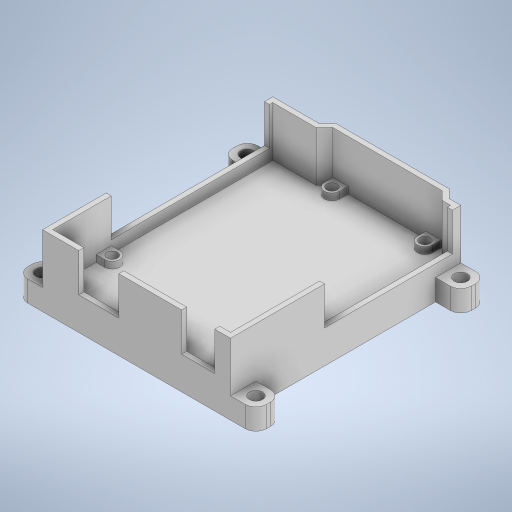
# Autodesk Inventor part: ArduinoCaseBottom
Saved by Autodesk Inventor 2024 (Build 280153000, 153)
## iProperties
Created: 2023-09-08
Part Number: ArduinoCaseBottom
Material: Generic
Document SubType Name: Modeling
Designer: 18179
Density: 1 g/cm^3
Appearance: Default
Autodesk Inventor part; units mm, degrees
(part 1 of 2)
ref_plane "YZ Plane" through (0, 0, 0) normal (1, 0, 0) x (0, 1, 0)
ref_plane "XZ Plane" through (0, 0, 0) normal (0, 1, 0) x (-1, 0, 0)
ref_plane "XY Plane" through (0, 0, 0) normal (0, 0, 1) x (1, 0, 0)
sketch "0" plane through (0, 0, 0) normal (0, 0, 1) x (1, 0, 0)
  line L0 (50.34, 19.545) -> (50.34, 17.135)
  line L1 (50.34, 17.135) -> (70.66, 17.135)
  line L2 (70.66, 17.135) -> (70.66, 19.545)
  line L3 (70.66, 19.545) -> (50.34, 19.545)
  line L4 (52.61, 19.34) -> (52.61, 17.34)
  line L5 (52.61, 17.34) -> (50.61, 17.34)
  line L6 (50.61, 17.34) -> (50.61, 19.34)
  line L7 (50.61, 19.34) -> (52.61, 19.34)
  line L8 (55.15, 17.34) -> (53.15, 17.34)
  line L9 (53.15, 17.34) -> (53.15, 19.34)
  line L10 (53.15, 19.34) -> (55.15, 19.34)
  line L11 (55.15, 19.34) -> (55.15, 17.34)
  line L12 (55.69, 17.34) -> (55.69, 19.34)
  line L13 (55.69, 19.34) -> (57.69, 19.34)
  line L14 (57.69, 19.34) -> (57.69, 17.34)
  line L15 (57.69, 17.34) -> (55.69, 17.34)
  line L16 (58.23, 17.34) -> (58.23, 19.34)
  line L17 (58.23, 19.34) -> (60.23, 19.34)
  line L18 (60.23, 19.34) -> (60.23, 17.34)
  line L19 (60.23, 17.34) -> (58.23, 17.34)
  line L20 (60.77, 17.34) -> (60.77, 19.34)
  line L21 (60.77, 19.34) -> (62.77, 19.34)
  line L22 (62.77, 19.34) -> (62.77, 17.34)
  line L23 (62.77, 17.34) -> (60.77, 17.34)
  line L24 (63.31, 17.34) -> (63.31, 19.34)
  line L25 (63.31, 19.34) -> (65.31, 19.34)
  line L26 (65.31, 19.34) -> (65.31, 17.34)
  line L27 (65.31, 17.34) -> (63.31, 17.34)
  line L28 (65.85, 17.34) -> (65.85, 19.34)
  line L29 (65.85, 19.34) -> (67.85, 19.34)
  line L30 (67.85, 19.34) -> (67.85, 17.34)
  line L31 (67.85, 17.34) -> (65.85, 17.34)
  line L32 (68.39, 17.34) -> (68.39, 19.34)
  line L33 (68.39, 19.34) -> (70.39, 19.34)
  line L34 (70.39, 19.34) -> (70.39, 17.34)
  line L35 (70.39, 17.34) -> (68.39, 17.34)
  line L36 (23.416, 19.545) -> (23.416, 17.135)
  line L37 (23.416, 17.135) -> (48.816, 17.135)
  line L38 (48.816, 17.135) -> (48.816, 19.545)
  line L39 (48.816, 19.545) -> (23.416, 19.545)
  line L40 (25.686, 19.34) -> (25.686, 17.34)
  line L41 (25.686, 17.34) -> (23.686, 17.34)
  line L42 (23.686, 17.34) -> (23.686, 19.34)
  line L43 (23.686, 19.34) -> (25.686, 19.34)
  line L44 (28.226, 17.34) -> (26.226, 17.34)
  line L45 (26.226, 17.34) -> (26.226, 19.34)
  line L46 (26.226, 19.34) -> (28.226, 19.34)
  line L47 (28.226, 19.34) -> (28.226, 17.34)
  line L48 (28.766, 17.34) -> (28.766, 19.34)
  line L49 (28.766, 19.34) -> (30.766, 19.34)
  line L50 (30.766, 19.34) -> (30.766, 17.34)
  line L51 (30.766, 17.34) -> (28.766, 17.34)
  line L52 (31.306, 17.34) -> (31.306, 19.34)
  line L53 (31.306, 19.34) -> (33.306, 19.34)
  line L54 (33.306, 19.34) -> (33.306, 17.34)
  line L55 (33.306, 17.34) -> (31.306, 17.34)
  line L56 (33.846, 17.34) -> (33.846, 19.34)
  line L57 (33.846, 19.34) -> (35.846, 19.34)
  line L58 (35.846, 19.34) -> (35.846, 17.34)
  line L59 (35.846, 17.34) -> (33.846, 17.34)
  line L60 (36.386, 17.34) -> (36.386, 19.34)
  line L61 (36.386, 19.34) -> (38.386, 19.34)
  line L62 (38.386, 19.34) -> (38.386, 17.34)
  line L63 (38.386, 17.34) -> (36.386, 17.34)
  line L64 (38.926, 17.34) -> (38.926, 19.34)
  line L65 (38.926, 19.34) -> (40.926, 19.34)
  line L66 (40.926, 19.34) -> (40.926, 17.34)
  line L67 (40.926, 17.34) -> (38.926, 17.34)
  line L68 (41.466, 17.34) -> (41.466, 19.34)
  line L69 (41.466, 19.34) -> (43.466, 19.34)
  line L70 (43.466, 19.34) -> (43.466, 17.34)
  line L71 (43.466, 17.34) -> (41.466, 17.34)
  line L72 (44.006, 17.34) -> (44.006, 19.34)
  line L73 (44.006, 19.34) -> (46.006, 19.34)
  line L74 (46.006, 19.34) -> (46.006, 17.34)
  line L75 (46.006, 17.34) -> (44.006, 17.34)
  line L76 (46.546, 17.34) -> (46.546, 19.34)
  line L77 (46.546, 19.34) -> (48.546, 19.34)
  line L78 (48.546, 19.34) -> (48.546, 17.34)
  line L79 (48.546, 17.34) -> (46.546, 17.34)
  line L80 (0, 0) -> (15.58, 0)
  line L81 (15.58, 0) -> (15.58, 11.12)
  line L82 (15.58, 11.12) -> (0, 11.12)
  line L83 (0, 11.12) -> (0, 0)
  line L84 (32.56, -28.715) -> (32.56, -31.125)
  line L85 (32.56, -31.125) -> (52.88, -31.125)
  line L86 (52.88, -31.125) -> (52.88, -28.715)
  line L87 (52.88, -28.715) -> (32.56, -28.715)
  line L88 (34.83, -28.92) -> (34.83, -30.92)
  line L89 (34.83, -30.92) -> (32.83, -30.92)
  line L90 (32.83, -30.92) -> (32.83, -28.92)
  line L91 (32.83, -28.92) -> (34.83, -28.92)
  line L92 (37.37, -30.92) -> (35.37, -30.92)
  line L93 (35.37, -30.92) -> (35.37, -28.92)
  line L94 (35.37, -28.92) -> (37.37, -28.92)
  line L95 (37.37, -28.92) -> (37.37, -30.92)
  line L96 (37.91, -30.92) -> (37.91, -28.92)
  line L97 (37.91, -28.92) -> (39.91, -28.92)
  line L98 (39.91, -28.92) -> (39.91, -30.92)
  line L99 (39.91, -30.92) -> (37.91, -30.92)
  line L100 (40.45, -30.92) -> (40.45, -28.92)
  line L101 (40.45, -28.92) -> (42.45, -28.92)
  line L102 (42.45, -28.92) -> (42.45, -30.92)
  line L103 (42.45, -30.92) -> (40.45, -30.92)
  line L104 (42.99, -30.92) -> (42.99, -28.92)
  line L105 (42.99, -28.92) -> (44.99, -28.92)
  line L106 (44.99, -28.92) -> (44.99, -30.92)
  line L107 (44.99, -30.92) -> (42.99, -30.92)
  line L108 (45.53, -30.92) -> (45.53, -28.92)
  line L109 (45.53, -28.92) -> (47.53, -28.92)
  line L110 (47.53, -28.92) -> (47.53, -30.92)
  line L111 (47.53, -30.92) -> (45.53, -30.92)
  line L112 (48.07, -30.92) -> (48.07, -28.92)
  line L113 (48.07, -28.92) -> (50.07, -28.92)
  line L114 (50.07, -28.92) -> (50.07, -30.92)
  line L115 (50.07, -30.92) -> (48.07, -30.92)
  line L116 (50.61, -30.92) -> (50.61, -28.92)
  line L117 (50.61, -28.92) -> (52.61, -28.92)
  line L118 (52.61, -28.92) -> (52.61, -30.92)
  line L119 (52.61, -30.92) -> (50.61, -30.92)
  line L120 (55.42, -28.715) -> (55.42, -31.125)
  line L121 (55.42, -31.125) -> (70.66, -31.125)
  line L122 (70.66, -31.125) -> (70.66, -28.715)
  line L123 (70.66, -28.715) -> (55.42, -28.715)
  line L124 (57.69, -28.92) -> (57.69, -30.92)
  line L125 (57.69, -30.92) -> (55.69, -30.92)
  line L126 (55.69, -30.92) -> (55.69, -28.92)
  line L127 (55.69, -28.92) -> (57.69, -28.92)
  line L128 (60.23, -30.92) -> (58.23, -30.92)
  line L129 (58.23, -30.92) -> (58.23, -28.92)
  line L130 (58.23, -28.92) -> (60.23, -28.92)
  line L131 (60.23, -28.92) -> (60.23, -30.92)
  line L132 (60.77, -30.92) -> (60.77, -28.92)
  line L133 (60.77, -28.92) -> (62.77, -28.92)
  line L134 (62.77, -28.92) -> (62.77, -30.92)
  line L135 (62.77, -30.92) -> (60.77, -30.92)
  line L136 (63.31, -30.92) -> (63.31, -28.92)
  line L137 (63.31, -28.92) -> (65.31, -28.92)
  line L138 (65.31, -28.92) -> (65.31, -30.92)
  line L139 (65.31, -30.92) -> (63.31, -30.92)
  line L140 (65.85, -30.92) -> (65.85, -28.92)
  line L141 (65.85, -28.92) -> (67.85, -28.92)
  line L142 (67.85, -28.92) -> (67.85, -30.92)
  line L143 (67.85, -30.92) -> (65.85, -30.92)
  line L144 (68.39, -30.92) -> (68.39, -28.92)
  line L145 (68.39, -28.92) -> (70.39, -28.92)
  line L146 (70.39, -28.92) -> (70.39, -30.92)
  line L147 (70.39, -30.92) -> (68.39, -30.92)
  arc A0 (68.8, -0.76) -> (68.3, -1.26) centre (68.8, -1.26) ccw
  line L148 (68.3, -1.26) -> (68.3, -2.8)
  arc A1 (68.3, -2.8) -> (68.8, -3.3) centre (68.8, -2.8) ccw
  line L149 (68.8, -3.3) -> (72.8, -3.3)
  arc A2 (72.8, -3.3) -> (73.3, -2.8) centre (72.8, -2.8) ccw
  line L150 (73.3, -2.8) -> (73.3, -1.26)
  arc A3 (73.3, -1.26) -> (72.8, -0.76) centre (72.8, -1.26) ccw
  line L151 (72.8, -0.76) -> (68.8, -0.76)
  line L152 (69.905, -2.405) -> (69.155, -2.405)
  line L153 (69.155, -2.405) -> (69.155, -1.655)
  line L154 (69.155, -1.655) -> (69.905, -1.655)
  line L155 (69.905, -1.655) -> (69.905, -2.405)
  line L156 (72.445, -2.405) -> (71.695, -2.405)
  line L157 (71.695, -2.405) -> (71.695, -1.655)
  line L158 (71.695, -1.655) -> (72.445, -1.655)
  line L159 (72.445, -1.655) -> (72.445, -2.405)
  arc A4 (68.8, -3.3) -> (68.3, -3.8) centre (68.8, -3.8) ccw
  line L160 (68.3, -3.8) -> (68.3, -5.34)
  arc A5 (68.3, -5.34) -> (68.8, -5.84) centre (68.8, -5.34) ccw
  line L161 (68.8, -5.84) -> (72.8, -5.84)
  arc A6 (72.8, -5.84) -> (73.3, -5.34) centre (72.8, -5.34) ccw
  line L162 (73.3, -5.34) -> (73.3, -3.8)
  arc A7 (73.3, -3.8) -> (72.8, -3.3) centre (72.8, -3.8) ccw
  line L163 (72.8, -3.3) -> (68.8, -3.3)
  line L164 (69.905, -4.945) -> (69.155, -4.945)
  line L165 (69.155, -4.945) -> (69.155, -4.195)
  line L166 (69.155, -4.195) -> (69.905, -4.195)
  line L167 (69.905, -4.195) -> (69.905, -4.945)
  line L168 (72.445, -4.945) -> (71.695, -4.945)
  line L169 (71.695, -4.945) -> (71.695, -4.195)
  line L170 (71.695, -4.195) -> (72.445, -4.195)
  line L171 (72.445, -4.195) -> (72.445, -4.945)
  arc A8 (68.8, -5.84) -> (68.3, -6.34) centre (68.8, -6.34) ccw
  line L172 (68.3, -6.34) -> (68.3, -7.88)
  arc A9 (68.3, -7.88) -> (68.8, -8.38) centre (68.8, -7.88) ccw
  line L173 (68.8, -8.38) -> (72.8, -8.38)
  arc A10 (72.8, -8.38) -> (73.3, -7.88) centre (72.8, -7.88) ccw
  line L174 (73.3, -7.88) -> (73.3, -6.34)
  arc A11 (73.3, -6.34) -> (72.8, -5.84) centre (72.8, -6.34) ccw
  line L175 (72.8, -5.84) -> (68.8, -5.84)
  line L176 (69.905, -7.485) -> (69.155, -7.485)
  line L177 (69.155, -7.485) -> (69.155, -6.735)
  line L178 (69.155, -6.735) -> (69.905, -6.735)
  line L179 (69.905, -6.735) -> (69.905, -7.485)
  line L180 (72.445, -7.485) -> (71.695, -7.485)
  line L181 (71.695, -7.485) -> (71.695, -6.735)
  line L182 (71.695, -6.735) -> (72.445, -6.735)
  line L183 (72.445, -6.735) -> (72.445, -7.485)
  arc A12 (20.37, 11.77) -> (20.87, 11.27) centre (20.87, 11.77) ccw
  line L184 (20.87, 11.27) -> (22.41, 11.27)
  arc A13 (22.41, 11.27) -> (22.91, 11.77) centre (22.41, 11.77) ccw
  line L185 (22.91, 11.77) -> (22.91, 15.77)
  arc A14 (22.91, 15.77) -> (22.41, 16.27) centre (22.41, 15.77) ccw
  line L186 (22.41, 16.27) -> (20.87, 16.27)
  arc A15 (20.87, 16.27) -> (20.37, 15.77) centre (20.87, 15.77) ccw
  line L187 (20.37, 15.77) -> (20.37, 11.77)
  line L188 (22.015, 12.875) -> (22.015, 12.125)
  line L189 (22.015, 12.125) -> (21.265, 12.125)
  line L190 (21.265, 12.125) -> (21.265, 12.875)
  line L191 (21.265, 12.875) -> (22.015, 12.875)
  line L192 (22.015, 15.415) -> (22.015, 14.665)
  line L193 (22.015, 14.665) -> (21.265, 14.665)
  line L194 (21.265, 14.665) -> (21.265, 15.415)
  line L195 (21.265, 15.415) -> (22.015, 15.415)
  arc A16 (25.45, 11.77) -> (25.95, 11.27) centre (25.95, 11.77) ccw
  line L196 (25.95, 11.27) -> (27.49, 11.27)
  arc A17 (27.49, 11.27) -> (27.99, 11.77) centre (27.49, 11.77) ccw
  line L197 (27.99, 11.77) -> (27.99, 15.77)
  arc A18 (27.99, 15.77) -> (27.49, 16.27) centre (27.49, 15.77) ccw
  line L198 (27.49, 16.27) -> (25.95, 16.27)
  arc A19 (25.95, 16.27) -> (25.45, 15.77) centre (25.95, 15.77) ccw
  line L199 (25.45, 15.77) -> (25.45, 11.77)
  line L200 (27.095, 12.875) -> (27.095, 12.125)
  line L201 (27.095, 12.125) -> (26.345, 12.125)
  line L202 (26.345, 12.125) -> (26.345, 12.875)
  line L203 (26.345, 12.875) -> (27.095, 12.875)
  line L204 (27.095, 15.415) -> (27.095, 14.665)
  line L205 (27.095, 14.665) -> (26.345, 14.665)
  line L206 (26.345, 14.665) -> (26.345, 15.415)
  line L207 (26.345, 15.415) -> (27.095, 15.415)
  arc A20 (22.91, 11.77) -> (23.41, 11.27) centre (23.41, 11.77) ccw
  line L208 (23.41, 11.27) -> (24.95, 11.27)
  arc A21 (24.95, 11.27) -> (25.45, 11.77) centre (24.95, 11.77) ccw
  line L209 (25.45, 11.77) -> (25.45, 15.77)
  arc A22 (25.45, 15.77) -> (24.95, 16.27) centre (24.95, 15.77) ccw
  line L210 (24.95, 16.27) -> (23.41, 16.27)
  arc A23 (23.41, 16.27) -> (22.91, 15.77) centre (23.41, 15.77) ccw
  line L211 (22.91, 15.77) -> (22.91, 11.77)
  line L212 (24.555, 12.875) -> (24.555, 12.125)
  line L213 (24.555, 12.125) -> (23.805, 12.125)
  line L214 (23.805, 12.125) -> (23.805, 12.875)
  line L215 (23.805, 12.875) -> (24.555, 12.875)
  line L216 (24.555, 15.415) -> (24.555, 14.665)
  line L217 (24.555, 14.665) -> (23.805, 14.665)
  line L218 (23.805, 14.665) -> (23.805, 15.415)
  line L219 (23.805, 15.415) -> (24.555, 15.415)
  line L220 (64.91, 3.516) -> (64.91, 4.716)
  line L221 (64.91, 4.716) -> (63.71, 4.716)
  line L222 (63.71, 4.716) -> (63.71, 3.516)
  line L223 (63.71, 3.516) -> (64.91, 3.516)
  line L224 (34.43, 8.977) -> (34.43, 10.177)
  line L225 (34.43, 10.177) -> (33.23, 10.177)
  line L226 (33.23, 10.177) -> (33.23, 8.977)
  line L227 (33.23, 8.977) -> (34.43, 8.977)
  line L228 (34.43, 3.77) -> (34.43, 4.97)
  line L229 (34.43, 4.97) -> (33.23, 4.97)
  line L230 (33.23, 4.97) -> (33.23, 3.77)
  line L231 (33.23, 3.77) -> (34.43, 3.77)
  line L232 (34.43, 1.23) -> (34.43, 2.43)
  line L233 (34.43, 2.43) -> (33.23, 2.43)
  line L234 (33.23, 2.43) -> (33.23, 1.23)
  line L235 (33.23, 1.23) -> (34.43, 1.23)
  line L236 (5.89, -32.46) -> (71.93, -32.46)
  line L237 (71.93, -32.46) -> (71.93, -29.92)
  line L238 (71.93, -29.92) -> (74.47, -27.38)
  line L239 (74.47, -27.38) -> (74.47, 5.386)
  line L240 (74.47, 5.386) -> (71.93, 7.926)
  line L241 (71.93, 7.926) -> (71.93, 20.88)
  line L242 (71.93, 20.88) -> (5.89, 20.88)
  line L243 (5.89, 20.88) -> (5.89, -32.46)
  line L244 (15.985, -20.785) -> (7.485, -20.785)
  line L245 (7.485, -20.785) -> (7.485, -20.285)
  line L246 (7.485, -20.285) -> (3.985, -20.285)
  line L247 (3.985, -29.285) -> (7.485, -29.285)
  line L248 (7.485, -29.285) -> (7.485, -28.785)
  line L249 (7.485, -28.785) -> (15.985, -28.785)
  line L250 (15.48, 11.58) -> (0.1, 11.58)
  line L251 (16.04, 0) -> (16.04, 11.12)
  line L252 (0.1, -0.46) -> (15.48, -0.46)
  line L253 (-0.46, 0) -> (-0.46, 11.12)
  circle A24 centre (12.24, 16.943) radius 1.5
  line L254 (17.685, -20.785) -> (17.685, -28.785)
  line L255 (3.985, -20.785) -> (3.985, -28.785)
  circle A25 centre (21.13, 18.34) radius 1.5875
  circle A26 centre (19.86, -29.92) radius 1.5875
  circle A27 centre (71.93, 3.1) radius 1.5875
  circle A28 centre (71.93, -24.84) radius 1.5875
  circle A29 centre (68.755, -19.887) radius 0.4
  circle A30 centre (68.755, -12.267) radius 0.4
  circle A31 centre (66.215, -19.887) radius 0.4
  circle A32 centre (66.215, -12.267) radius 0.4
  circle A33 centre (63.675, -19.887) radius 0.4
  circle A34 centre (63.675, -12.267) radius 0.4
  circle A35 centre (61.135, -19.887) radius 0.4
  circle A36 centre (61.135, -12.267) radius 0.4
  circle A37 centre (58.595, -19.887) radius 0.4
  circle A38 centre (58.595, -12.267) radius 0.4
  circle A39 centre (56.055, -19.887) radius 0.4
  circle A40 centre (56.055, -12.267) radius 0.4
  circle A41 centre (53.515, -19.887) radius 0.4
  circle A42 centre (53.515, -12.267) radius 0.4
  circle A43 centre (50.975, -19.887) radius 0.4
  circle A44 centre (50.975, -12.267) radius 0.4
  circle A45 centre (48.435, -19.887) radius 0.4
  circle A46 centre (48.435, -12.267) radius 0.4
  circle A47 centre (45.895, -19.887) radius 0.4
  circle A48 centre (45.895, -12.267) radius 0.4
  circle A49 centre (43.355, -19.887) radius 0.4
  circle A50 centre (43.355, -12.267) radius 0.4
  circle A51 centre (40.815, -19.887) radius 0.4
  circle A52 centre (40.815, -12.267) radius 0.4
  circle A53 centre (38.275, -19.887) radius 0.4
  circle A54 centre (38.275, -12.267) radius 0.4
  circle A55 centre (35.735, -19.887) radius 0.4
  circle A56 centre (35.735, -12.267) radius 0.4
  circle A57 centre (22.273, -6.298) radius 0.5
  circle A58 centre (27.353, -6.298) radius 0.5
  circle A59 centre (24.178, 7.418) radius 0.4
  circle A60 centre (26.718, 7.418) radius 0.4
  circle A61 centre (26.718, 9.958) radius 0.4
  circle A62 centre (24.178, 9.958) radius 0.4
  circle A63 centre (21.638, 12.498) radius 0.4
  circle A64 centre (24.178, 12.498) radius 0.4
  circle A65 centre (26.718, 12.498) radius 0.4
  circle A66 centre (26.718, 15.038) radius 0.4
  circle A67 centre (24.178, 15.038) radius 0.4
  circle A68 centre (21.638, 15.038) radius 0.4
  circle A69 centre (69.53, -2.03) radius 0.4
  circle A70 centre (69.53, -4.57) radius 0.4
  circle A71 centre (69.53, -7.11) radius 0.4
  circle A72 centre (72.07, -7.11) radius 0.4
  circle A73 centre (72.07, -4.57) radius 0.4
  circle A74 centre (72.07, -2.03) radius 0.4
  circle A75 centre (54.15, 18.34) radius 0.4
  circle A76 centre (27.226, 18.34) radius 0.4
  circle A77 centre (51.61, 18.34) radius 0.4
  circle A78 centre (36.37, -29.92) radius 0.4
  circle A79 centre (24.686, 18.34) radius 0.4
  circle A80 centre (33.83, -29.92) radius 0.4
  circle A81 centre (21.13, 18.34) radius 1.5875
  circle A82 centre (19.86, -29.92) radius 1.5875
  circle A83 centre (71.93, 3.1) radius 1.5875
  circle A84 centre (71.93, -24.84) radius 1.5875
  circle A85 centre (38.91, -29.92) radius 0.4
  circle A86 centre (41.45, -29.92) radius 0.4
  circle A87 centre (43.99, -29.92) radius 0.4
  circle A88 centre (46.53, -29.92) radius 0.4
  circle A89 centre (49.07, -29.92) radius 0.4
  circle A90 centre (51.61, -29.92) radius 0.4
  circle A91 centre (56.69, -29.92) radius 0.4
  circle A92 centre (59.23, -29.92) radius 0.4
  circle A93 centre (61.77, -29.92) radius 0.4
  circle A94 centre (64.31, -29.92) radius 0.4
  circle A95 centre (66.85, -29.92) radius 0.4
  circle A96 centre (69.39, -29.92) radius 0.4
  circle A97 centre (29.766, 18.34) radius 0.4
  circle A98 centre (32.306, 18.34) radius 0.4
  circle A99 centre (34.846, 18.34) radius 0.4
  circle A100 centre (37.386, 18.34) radius 0.4
  circle A101 centre (39.926, 18.34) radius 0.4
  circle A102 centre (42.466, 18.34) radius 0.4
  circle A103 centre (45.006, 18.34) radius 0.4
  circle A104 centre (47.546, 18.34) radius 0.4
  circle A105 centre (56.69, 18.34) radius 0.4
  circle A106 centre (59.23, 18.34) radius 0.4
  circle A107 centre (61.77, 18.34) radius 0.4
  circle A108 centre (64.31, 18.34) radius 0.4
  circle A109 centre (66.85, 18.34) radius 0.4
  circle A110 centre (69.39, 18.34) radius 0.4
  line L256 (4.3025, 20.88) -> (4.3025, -32.46)
  line L257 (71.93, 22.4675) -> (5.89, 22.4675)
  line L258 (73.5175, 7.926) -> (73.5175, 20.88)
  line L259 (75.5925, 6.5085) -> (73.0525, 9.0485)
  line L260 (76.0575, -27.38) -> (76.0575, 5.386)
  line L261 (73.0525, -31.0425) -> (75.5925, -28.5025)
  line L262 (73.5175, -32.46) -> (73.5175, -29.92)
  line L263 (5.89, -34.0475) -> (71.93, -34.0475)
  line L264 (4.3025, 20.88) -> (4.3025, 22.4675)
  line L265 (4.3025, 22.4675) -> (5.89, 22.4675)
  line L266 (71.93, 22.4675) -> (73.5175, 22.4675)
  line L267 (73.5175, 22.4675) -> (73.5175, 20.88)
  line L268 (76.0575, 5.386) -> (76.0575, 7.7785)
  line L269 (75.5925, 6.5085) -> (76.0575, 6.0436)
  line L270 (71.93, -34.0475) -> (73.5175, -34.0475)
  line L271 (73.5175, -34.0475) -> (73.5175, -32.46)
  line L272 (75.5925, -28.5025) -> (76.6188, -27.4763)
  line L273 (76.0575, -27.38) -> (76.1056, -27.9894)
  line L274 (4.3025, -32.46) -> (4.3025, -34.0475)
  line L275 (4.3025, -34.0475) -> (5.89, -34.0475)
  line L276 (4.3025, 22.4675) -> (11.9225, 22.4675)
  line L277 (11.9225, 22.4675) -> (11.9225, 26.9125)
  line L278 (8.7475, 30.0875) -> (7.4775, 30.0875)
  line L279 (4.3025, 26.9125) -> (4.3025, 22.4675)
  circle A111 centre (8.1125, 26.2775) radius 2
  line L280 (73.5175, 22.4675) -> (65.8975, 22.4675)
  line L281 (65.8975, 22.4675) -> (65.8975, 26.9125)
  line L282 (69.0725, 30.0875) -> (70.3425, 30.0875)
  line L283 (73.5175, 26.9125) -> (73.5175, 22.4675)
  line L284 (4.3025, -34.0475) -> (11.9225, -34.0475)
  line L285 (11.9225, -34.0475) -> (11.9225, -38.4925)
  line L286 (8.7475, -41.6675) -> (7.4775, -41.6675)
  line L287 (4.3025, -38.4925) -> (4.3025, -34.0475)
  line L288 (73.5175, -34.0475) -> (65.8975, -34.0475)
  line L289 (65.8975, -34.0475) -> (65.8975, -38.4925)
  line L290 (69.0725, -41.6675) -> (70.3425, -41.6675)
  line L291 (73.5175, -38.4925) -> (73.5175, -34.0475)
  circle A112 centre (8.1125, -37.8575) radius 2
  circle A113 centre (69.7075, -37.8575) radius 2
  circle A114 centre (69.7075, 26.2775) radius 2
  arc A115 (7.4775, 30.0875) -> (4.3025, 26.9125) centre (7.4775, 26.9125) ccw
  arc A116 (11.9225, 26.9125) -> (8.7475, 30.0875) centre (8.7475, 26.9125) ccw
  arc A117 (69.0725, 30.0875) -> (65.8975, 26.9125) centre (69.0725, 26.9125) ccw
  arc A118 (73.5175, 26.9125) -> (70.3425, 30.0875) centre (70.3425, 26.9125) ccw
  arc A119 (70.3425, -41.6675) -> (73.5175, -38.4925) centre (70.3425, -38.4925) ccw
  arc A120 (65.8975, -38.4925) -> (69.0725, -41.6675) centre (69.0725, -38.4925) ccw
  arc A121 (8.7475, -41.6675) -> (11.9225, -38.4925) centre (8.7475, -38.4925) ccw
  arc A122 (4.3025, -38.4925) -> (7.4775, -41.6675) centre (7.4775, -38.4925) ccw
  point P0 (11.9225, 30.0875)
  point P1 (4.3025, 30.0875)
  point P2 (65.8975, 30.0875)
  point P3 (73.5175, 30.0875)
  point P4 (11.9225, -41.6675)
  point P5 (4.3025, -41.6675)
  point P6 (65.8975, -41.6675)
  point P7 (73.5175, -41.6675)
  point P8 (4.3025, 11.12)
  point P9 (4.3025, 0)
  point P10 (5.89, 0)
  point P11 (5.89, 11.12)
  point P12 (4.3025, 11.58)
  point P13 (5.89, 11.58)
  point P14 (74.47, 5.386)
  point P15 (5.89, -32.46)
  point P16 (5.89, -0.46)
  point P17 (4.3025, -0.46)
  point P18 (73.5175, -30.5776)
  point P19 (73.5175, 8.5836)
  point P20 (4.3025, -20.285)
  point P21 (4.3025, -29.285)
  point P22 (5.89, -29.285)
  point P23 (5.89, -20.285)
  point P24 (69.905, -4.7092)
  point P25 (69.6692, -4.945)
  point P26 (69.3908, -4.945)
  point P27 (69.155, -4.7092)
  point P28 (69.155, -4.4308)
  point P29 (69.3908, -4.195)
  point P30 (69.6692, -4.195)
  point P31 (69.905, -4.4308)
  point P32 (72.445, -4.7092)
  point P33 (72.2092, -4.945)
  point P34 (71.9308, -4.945)
  point P35 (71.695, -4.7092)
  point P36 (71.695, -4.4308)
  point P37 (71.9308, -4.195)
  point P38 (72.2092, -4.195)
  point P39 (72.445, -4.4308)
  point P40 (69.905, -7.2492)
  point P41 (69.6692, -7.485)
  point P42 (69.3908, -7.485)
  point P43 (69.155, -7.2492)
  point P44 (69.155, -6.9708)
  point P45 (69.3908, -6.735)
  point P46 (69.6692, -6.735)
  point P47 (69.905, -6.9708)
  point P48 (68.8, -0.76)
  point P49 (68.3, -6.34)
  point P50 (68.8, -8.38)
  point P51 (69.905, -2.1692)
  point P52 (69.6692, -2.405)
  point P53 (69.3908, -2.405)
  point P54 (69.155, -2.1692)
  point P55 (69.155, -1.8908)
  point P56 (69.3908, -1.655)
  point P57 (69.6692, -1.655)
  point P58 (69.905, -1.8908)
  point P59 (72.445, -2.1692)
  point P60 (72.2092, -2.405)
  point P61 (71.9308, -2.405)
  point P62 (71.695, -2.1692)
  point P63 (71.695, -1.8908)
  point P64 (71.9308, -1.655)
  point P65 (72.2092, -1.655)
  point P66 (72.445, -1.8908)
  point P67 (24.555, 12.3643)
  point P68 (24.3225, 12.125)
  point P69 (24.0335, 12.125)
  point P70 (23.805, 12.3535)
  point P71 (23.805, 12.6425)
  point P72 (24.0443, 12.875)
  point P73 (24.3117, 12.875)
  point P74 (24.555, 12.6317)
  point P75 (24.555, 14.9043)
  point P76 (24.3225, 14.665)
  point P77 (24.0335, 14.665)
  point P78 (23.805, 14.8935)
  point P79 (23.805, 15.1825)
  point P80 (24.0443, 15.415)
  point P81 (24.3117, 15.415)
  point P82 (24.555, 15.1717)
  point P83 (27.095, 12.3643)
  point P84 (26.8625, 12.125)
  point P85 (26.5735, 12.125)
  point P86 (26.345, 12.3535)
  point P87 (26.345, 12.6425)
  point P88 (26.5843, 12.875)
  point P89 (26.8517, 12.875)
  point P90 (27.095, 12.6317)
  point P91 (27.095, 14.9043)
  point P92 (26.8625, 14.665)
  point P93 (26.5735, 14.665)
  point P94 (26.345, 14.8935)
  point P95 (26.345, 15.1825)
  point P96 (26.5843, 15.415)
  point P97 (26.8517, 15.415)
  point P98 (27.095, 15.1717)
  point P99 (22.41, 16.27)
  point P100 (20.37, 11.77)
  point P101 (23.41, 11.27)
  point P102 (27.49, 16.27)
  point P103 (24.95, 16.27)
  point P104 (22.015, 12.3643)
  point P105 (21.7825, 12.125)
  point P106 (21.4935, 12.125)
  point P107 (21.265, 12.3535)
  point P108 (21.265, 12.6425)
  point P109 (21.5043, 12.875)
  point P110 (21.7717, 12.875)
  point P111 (22.015, 12.6317)
  point P112 (22.015, 14.9043)
  point P113 (21.7825, 14.665)
  point P114 (21.4935, 14.665)
  point P115 (21.265, 14.8935)
  point P116 (21.265, 15.1825)
  point P117 (21.5043, 15.415)
  point P118 (21.7717, 15.415)
  point P119 (22.015, 15.1717)
  dimension "d0" = 1.5875
  dimension "d1" = 1.5875
  dimension "d2" = 1.5875
  dimension "d3" = 1.5875
  dimension "d4" = 1.5875
  dimension "d5" = 1.5875
  dimension "d6" = 1.5875
  dimension "d7" = 1.5875
  dimension "d8" = 7.62
  dimension "d9" = 7.62
  dimension "d10" = 4
  dimension "d11" = 7.62
  dimension "d12" = 7.62
  dimension "d13" = 7.62
  dimension "d14" = 7.62
  dimension "d15" = 7.62
  dimension "d16" = 7.62
  dimension "d17" = 4
  dimension "d18" = 4
  dimension "d19" = 4
  dimension "d20" = 3.175
  constraints: 584 end point, 131 horizontal, 131 vertical, 123 centre point, 64 point on circle, 18 point on line, 16 parallel, 16 tangent, 9 perpendicular, 7 equal radius, 1 midpoint, 784 other
  measures "d0" distance between parallel lines of L243 L256
  measures "d1" distance between parallel lines of L242 L257
  measures "d2" distance between parallel lines of L241 L258
  measures "d3" distance between parallel lines of L240 L259
  measures "d4" distance between parallel lines of L239 L260
  measures "d5" distance between parallel lines of L238 L261
  measures "d6" distance between parallel lines of L237 L262
  measures "d7" distance between parallel lines of L236 L263
  measures "d8" distance of point (4.302, 30.087) point (11.922, 30.087)
  measures "d9" distance of point (11.922, 30.087) L276.end
  measures "d10" diameter of A111
  measures "d11" distance of point (65.897, 30.087) point (73.517, 30.087)
  measures "d12" distance of L280.end point (65.897, 30.087)
  measures "d13" distance of point (11.922, -41.668) point (4.302, -41.668)
  measures "d14" distance of L284.end point (11.922, -41.668)
  measures "d15" distance of point (73.517, -41.668) point (65.897, -41.668)
  measures "d16" distance of point (65.897, -41.668) L288.end
  measures "d17" diameter of A112
  measures "d18" diameter of A113
  measures "d19" diameter of A114
  measures "d20" radius of A115
extrude "Extrusion1" add sketch "0" along normal blind 3.175 contours L256 L82 L243 L80 | L252 L243 L246 L256 | L256 L264 L265 L257 L266 L267 L258 L259 L269 L268 L260 L273 L272 L261 L262 L271 L270 L263 L275 L274 L247 L243 L236 L237 L238 L239 L240 L241 L242 L250 | L246 L243 L247 L256 | L279 A115 L278 A116 L277 L257 L265 | L275 L263 L285 A121 L286 A122 L287 | L281 A117 L282 A118 L283 L266 L257 | L263 L270 L291 A119 L290 A120 L289
extrude "Extrusion2" add sketch "0" along normal blind 3.175 contours L80 L243 L252 L256 | L256 L250 L243 L82
sketch "Sketch3" plane through (0, 0, 3.175) normal (0, 0, 1) x (1, 0, 0)
  line L0 (4.3025, 26.9125) -> (4.3025, -38.4925) projected
  arc A0 (4.3025, -38.4925) -> (7.4775, -41.6675) centre (7.4775, -38.4925) ccw projected
  line L1 (7.4775, -41.6675) -> (8.7475, -41.6675) projected
  arc A1 (8.7475, -41.6675) -> (11.9225, -38.4925) centre (8.7475, -38.4925) ccw projected
  line L2 (11.9225, -38.4925) -> (11.9225, -34.0475) projected
  line L3 (11.9225, -34.0475) -> (65.8975, -34.0475) projected
  line L4 (65.8975, -34.0475) -> (65.8975, -38.4925) projected
  arc A2 (65.8975, -38.4925) -> (69.0725, -41.6675) centre (69.0725, -38.4925) ccw projected
  line L5 (69.0725, -41.6675) -> (70.3425, -41.6675) projected
  arc A3 (70.3425, -41.6675) -> (73.5175, -38.4925) centre (70.3425, -38.4925) ccw projected
  line L6 (73.5175, -38.4925) -> (73.5175, -30.5776) projected
  line L7 (73.5175, -30.5776) -> (76.1056, -27.9894) projected
  line L8 (76.1056, -27.9894) -> (76.0575, -27.38) projected
  line L9 (76.0575, -27.38) -> (76.0575, 6.0436) projected
  line L10 (76.0575, 6.0436) -> (73.5175, 8.5836) projected
  line L11 (73.5175, 8.5836) -> (73.5175, 26.9125) projected
  arc A4 (73.5175, 26.9125) -> (70.3425, 30.0875) centre (70.3425, 26.9125) ccw projected
  line L12 (70.3425, 30.0875) -> (69.0725, 30.0875) projected
  arc A5 (69.0725, 30.0875) -> (65.8975, 26.9125) centre (69.0725, 26.9125) ccw projected
  line L13 (65.8975, 26.9125) -> (65.8975, 22.4675) projected
  line L14 (65.8975, 22.4675) -> (11.9225, 22.4675) projected
  line L15 (11.9225, 22.4675) -> (11.9225, 26.9125) projected
  arc A6 (11.9225, 26.9125) -> (8.7475, 30.0875) centre (8.7475, 26.9125) ccw projected
  line L16 (8.7475, 30.0875) -> (7.4775, 30.0875) projected
  arc A7 (7.4775, 30.0875) -> (4.3025, 26.9125) centre (7.4775, 26.9125) ccw projected
  circle A8 centre (8.1125, 26.2775) radius 2 projected
  circle A9 centre (69.7075, 26.2775) radius 2 projected
  circle A10 centre (69.7075, -37.8575) radius 2 projected
  circle A11 centre (8.1125, -37.8575) radius 2 projected
  line L17 (5.89, -32.46) -> (5.89, 20.88) projected
  line L18 (5.89, 20.88) -> (71.93, 20.88) projected
  line L19 (71.93, 20.88) -> (71.93, 7.926) projected
  line L20 (71.93, 7.926) -> (74.47, 5.386) projected
  line L21 (74.47, 5.386) -> (74.47, -27.38) projected
  line L22 (74.47, -27.38) -> (71.93, -29.92) projected
  line L23 (71.93, -29.92) -> (71.93, -32.46) projected
  line L24 (71.93, -32.46) -> (5.89, -32.46) projected
  point P0 (0, 0)
extrude "Extrusion3" add sketch "Sketch3" along normal blind 3.175 contours A7 L16 A6 L15 L14 L13 A5 L12 A4 L11 L10 L9 L8 L7 L6 A3 L5 A2 L4 L3 L2 A1 L1 A0 L0 | L17 L18 L19 L20 L21 L22 L23 L24
extrude "Extrusion4" cut sketch "0" along normal through all contours A25 | A26 | A27 | A28
sketch "Sketch4" plane through (0, 0, 6.35) normal (0, 0, 1) x (1, 0, 0)
  circle A0 centre (71.93, 3.1) radius 1.5875 projected
  circle A1 centre (21.13, 18.34) radius 1.5875 projected
  circle A2 centre (71.93, -24.84) radius 1.5875 projected
  circle A3 centre (19.86, -29.92) radius 1.5875 projected
  arc A4 (4.3025, -38.4925) -> (7.4775, -41.6675) centre (7.4775, -38.4925) ccw projected
  line L0 (7.4775, -41.6675) -> (8.7475, -41.6675) projected
  arc A5 (8.7475, -41.6675) -> (11.9225, -38.4925) centre (8.7475, -38.4925) ccw projected
  line L1 (11.9225, -38.4925) -> (11.9225, -34.0475) projected
  line L2 (11.9225, -34.0475) -> (65.8975, -34.0475) projected
  line L3 (65.8975, -34.0475) -> (65.8975, -38.4925) projected
  arc A6 (65.8975, -38.4925) -> (69.0725, -41.6675) centre (69.0725, -38.4925) ccw projected
  line L4 (69.0725, -41.6675) -> (70.3425, -41.6675) projected
  arc A7 (70.3425, -41.6675) -> (73.5175, -38.4925) centre (70.3425, -38.4925) ccw projected
  line L5 (73.5175, -38.4925) -> (73.5175, -30.5776) projected
  line L6 (73.5175, -30.5776) -> (76.1056, -27.9894) projected
  line L7 (76.1056, -27.9894) -> (76.0575, -27.38) projected
  line L8 (76.0575, -27.38) -> (76.0575, 6.0436) projected
  line L9 (76.0575, 6.0436) -> (73.5175, 8.5836) projected
  line L10 (73.5175, 8.5836) -> (73.5175, 26.9125) projected
  arc A8 (73.5175, 26.9125) -> (70.3425, 30.0875) centre (70.3425, 26.9125) ccw projected
  line L11 (70.3425, 30.0875) -> (69.0725, 30.0875) projected
  arc A9 (69.0725, 30.0875) -> (65.8975, 26.9125) centre (69.0725, 26.9125) ccw projected
  line L12 (65.8975, 26.9125) -> (65.8975, 22.4675) projected
  line L13 (65.8975, 22.4675) -> (11.9225, 22.4675) projected
  line L14 (11.9225, 22.4675) -> (11.9225, 26.9125) projected
  arc A10 (11.9225, 26.9125) -> (8.7475, 30.0875) centre (8.7475, 26.9125) ccw projected
  line L15 (8.7475, 30.0875) -> (7.4775, 30.0875) projected
  arc A11 (7.4775, 30.0875) -> (4.3025, 26.9125) centre (7.4775, 26.9125) ccw projected
  line L16 (4.3025, 26.9125) -> (4.3025, -38.4925) projected
  circle A12 centre (8.1125, -37.8575) radius 2 projected
  circle A13 centre (69.7075, -37.8575) radius 2 projected
  circle A14 centre (69.7075, 26.2775) radius 2 projected
  circle A15 centre (8.1125, 26.2775) radius 2 projected
  line L17 (10.3985, 20.9435) -> (67.4215, 20.9435)
  line L18 (67.4215, 20.9435) -> (67.4215, 26.9125)
  arc A16 (69.0725, 28.5635) -> (67.4215, 26.9125) centre (69.0725, 26.9125) ccw
  line L19 (69.0725, 28.5635) -> (70.3425, 28.5635)
  arc A17 (71.9935, 26.9125) -> (70.3425, 28.5635) centre (70.3425, 26.9125) ccw
  line L20 (71.9935, 26.9125) -> (71.9935, 7.9523)
  line L21 (71.9935, 7.9523) -> (74.5335, 5.4123)
  line L22 (74.5335, 5.4123) -> (74.5335, -27.4063)
  line L23 (74.5335, -27.4063) -> (71.9935, -29.9463)
  line L24 (71.9935, -29.9463) -> (71.9935, -38.4925)
  arc A18 (70.3425, -40.1435) -> (71.9935, -38.4925) centre (70.3425, -38.4925) ccw
  line L25 (70.3425, -40.1435) -> (69.0725, -40.1435)
  arc A19 (67.4215, -38.4925) -> (69.0725, -40.1435) centre (69.0725, -38.4925) ccw
  line L26 (67.4215, -38.4925) -> (67.4215, -32.5235)
  line L27 (67.4215, -32.5235) -> (10.3985, -32.5235)
  line L28 (10.3985, -32.5235) -> (10.3985, -38.4925)
  arc A20 (8.7475, -40.1435) -> (10.3985, -38.4925) centre (8.7475, -38.4925) ccw
  line L29 (8.7475, -40.1435) -> (7.4775, -40.1435)
  arc A21 (5.8265, -38.4925) -> (7.4775, -40.1435) centre (7.4775, -38.4925) ccw
  line L30 (5.8265, -38.4925) -> (5.8265, 26.9125)
  arc A22 (7.4775, 28.5635) -> (5.8265, 26.9125) centre (7.4775, 26.9125) ccw
  line L31 (7.4775, 28.5635) -> (8.7475, 28.5635)
  arc A23 (10.3985, 26.9125) -> (8.7475, 28.5635) centre (8.7475, 26.9125) ccw
  line L32 (10.3985, 26.9125) -> (10.3985, 20.9435)
  line L33 (10.3985, 20.9435) -> (5.8265, 20.9435)
  line L34 (67.4215, 20.9435) -> (71.9935, 20.9435)
  line L35 (67.4215, -32.5235) -> (71.9935, -32.5235)
  line L36 (10.3985, -32.5235) -> (5.8265, -32.5235)
  line L37 (65.8975, 22.4675) -> (73.5175, 22.4675)
  line L38 (11.9225, 22.4675) -> (4.3025, 22.4675)
  line L39 (11.9225, -34.0475) -> (4.3025, -34.0475)
  line L40 (65.8975, -34.0475) -> (73.5175, -34.0475)
  point P0 (0, 0)
  dimension "d29" = 1.524
  constraints: 48 end point, 16 point on circle, 12 point on line, 8 centre point, 4 perpendicular, 23 other
  measures "d29" distance between parallel lines of L13 L17
extrude "Extrusion5" add sketch "Sketch4" along normal blind 15 contours L16 L38 L30 L39 | L30 L36 L28 L39 | L38 L32 L33 L30 | L28 L27 L26 L40 L2 L39 | L38 L13 L37 L18 L17 L32 | L35 L24 L40 L26 | L18 L37 L20 L34 | L24 L23 L22 L21 L20 L37 L10 L9 L8 L7 L6 L5 L40
extrude "Extrusion6" cut sketch "0" along normal through all contours L256 L82 L243 L80 | L246 L243 L247 L256
sketch "Sketch5" plane through (0, 0, 6.35) normal (0, 0, 1) x (1, 0, 0)
  circle A0 centre (19.86, -29.92) radius 1.5875 projected
  circle A1 centre (71.93, -24.84) radius 1.5875 projected
  circle A2 centre (21.13, 18.34) radius 1.5875 projected
  circle A3 centre (71.93, 3.1) radius 1.5875 projected
  line L0 (5.8265, 11.12) -> (5.89, 11.12) projected
  line L1 (5.89, 11.12) -> (5.89, 0) projected
  line L2 (5.89, 0) -> (5.8265, 0) projected
  line L3 (5.8265, 20.9435) -> (5.8265, 11.12) projected
  line L4 (5.8265, -20.285) -> (5.89, -20.285) projected
  line L5 (5.89, -20.285) -> (5.89, -29.285) projected
  line L6 (5.89, -29.285) -> (5.8265, -29.285) projected
  line L7 (5.8265, -29.285) -> (5.8265, -32.5235) projected
  line L8 (5.8265, -32.5235) -> (71.9935, -32.5235) projected
  line L9 (71.9935, -32.5235) -> (71.9935, -29.9463) projected
  line L10 (71.9935, -29.9463) -> (74.5335, -27.4063) projected
  line L11 (74.5335, -27.4063) -> (74.5335, 5.4123) projected
  line L12 (74.5335, 5.4123) -> (71.9935, 7.9523) projected
  line L13 (71.9935, 7.9523) -> (71.9935, 20.9435) projected
  line L14 (71.9935, 20.9435) -> (5.8265, 20.9435) projected
  line L15 (5.8265, 0) -> (5.8265, -20.285) projected
  circle A4 centre (21.13, 18.34) radius 2.286
  circle A5 centre (71.93, 3.1) radius 2.286
  circle A6 centre (71.93, -24.84) radius 2.286
  circle A7 centre (19.86, -29.92) radius 2.286
  line L16 (21.13, 18.34) -> (23.416, 18.34)
  line L17 (23.416, 18.34) -> (23.416, 20.9435)
  line L18 (23.416, 20.9435) -> (21.13, 20.9435)
  line L19 (21.13, 20.9435) -> (21.13, 18.34)
  line L20 (21.13, 20.9435) -> (18.844, 20.9435)
  line L21 (18.844, 20.9435) -> (18.844, 18.34)
  line L22 (18.844, 18.34) -> (21.13, 18.34)
  line L23 (21.13, 18.34) -> (21.13, 20.9435)
  line L24 (71.93, 5.386) -> (74.5335, 5.386)
  line L25 (74.5335, 5.386) -> (74.5335, 3.1)
  line L26 (74.5335, 3.1) -> (71.93, 3.1)
  line L27 (71.93, 3.1) -> (71.93, 5.386)
  line L28 (74.5335, 3.1) -> (71.93, 3.1)
  line L29 (71.93, 3.1) -> (71.93, 0.814)
  line L30 (71.93, 0.814) -> (74.5335, 0.814)
  line L31 (74.5335, 0.814) -> (74.5335, 3.1)
  line L32 (71.93, -24.84) -> (74.5335, -24.84)
  line L33 (74.5335, -24.84) -> (74.5335, -22.554)
  line L34 (74.5335, -22.554) -> (71.93, -22.554)
  line L35 (71.93, -22.554) -> (71.93, -24.84)
  line L36 (71.93, -24.84) -> (74.5335, -24.84)
  line L37 (74.5335, -24.84) -> (74.5335, -27.126)
  line L38 (74.5335, -27.126) -> (71.93, -27.126)
  line L39 (71.93, -27.126) -> (71.93, -24.84)
  line L40 (19.86, -29.92) -> (22.146, -29.92)
  line L41 (22.146, -29.92) -> (22.146, -32.5235)
  line L42 (22.146, -32.5235) -> (19.86, -32.5235)
  line L43 (19.86, -32.5235) -> (19.86, -29.92)
  line L44 (71.93, -32.46) -> (5.89, -32.46) projected
  line L45 (19.86, -29.92) -> (17.574, -29.92)
  line L46 (17.574, -29.92) -> (17.574, -32.46)
  line L47 (17.574, -32.46) -> (19.86, -32.46)
  line L48 (19.86, -32.46) -> (19.86, -29.92)
  line L49 (17.574, -32.46) -> (19.86, -32.46)
  line L50 (19.86, -32.46) -> (19.86, -32.5235)
  line L51 (19.86, -32.5235) -> (17.574, -32.5235)
  line L52 (17.574, -32.5235) -> (17.574, -32.46)
  point P0 (0, 0)
  point P1 (22.146, -32.46)
  dimension "d36" = 4.572
  dimension "d37" = 4.572
  dimension "d38" = 4.572
  dimension "d39" = 4.572
  constraints: 72 end point, 18 parallel, 9 horizontal, 9 perpendicular, 8 point on line, 4 coincident, 3 centre point, 2 point on circle, 3 other
  measures "d37" diameter of A5
  measures "d38" diameter of A6
  measures "d39" diameter of A7
extrude "Extrusion8" add sketch "Sketch5" along normal blind 2 contours L40 A7 L43 A0 | A0 L45 A7 L40 | A0 L43 A7 L45 | L41 L44 L43 A7 | A7 L43 L44 L46 | L38 A6 L32 L11 | L32 A6 L34 L11 | L39 A1 L32 A6 | A6 L35 A1 L39 | L32 A1 L35 A6 | L30 A5 L26 L11 | L26 A5 L24 L11 | L29 A3 L26 A5 | A5 L27 A3 L29 | L26 A3 L27 A5 | L14 L19 A4 L21 | L14 L17 A4 L19 | L22 A2 L16 A4 | A4 L19 A2 L22 | A4 L16 A2 L19